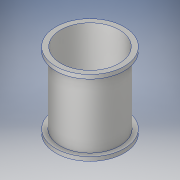
# Autodesk Inventor part: Radiation Sheild 55K
Saved by Autodesk Inventor 2018 (Build 220112000, 112)
## iProperties
Created: 2018-10-10
Part Number: Radiation Sheild 55K
Material: Aluminum 6061
Document SubType Name: Modeling
Designer: freyja
Mass: 27400.2 g
Surface Area: 12721.2 cm^2
Volume: 10148.2 cm^3
Density: 2.7 g/cm^3
Appearance: Aluminum - Flat
Author: freyja
Autodesk Inventor part; units mm, degrees
ref_plane "YZ Plane" through (0, 0, 0) normal (1, 0, 0) x (0, 1, 0)
ref_plane "XZ Plane" through (0, 0, 0) normal (0, 1, 0) x (-1, 0, 0)
ref_plane "XY Plane" through (0, 0, 0) normal (0, 0, 1) x (1, 0, 0)
sketch "Sketch1" plane through (0, 0, 0) normal (0, 1, 0) x (-1, 0, 0)
  circle A0 centre (0, 0) radius 184.15
  circle A1 centre (0, 0) radius 215.9
  dimension "d0" = 368.3
  dimension "d1" = 431.8
  constraints: 2 centre point, 2 coincident
  measures "d0" diameter of A0
  measures "d1" diameter of A1
extrude "Extrusion1" add sketch "Sketch1" along normal blind 25.4
sketch "Sketch2" plane through (0, 25.4, 0) normal (0, 1, 0) x (1, 0, 0)
  circle A0 centre (0, 0) radius 184.15
  circle A1 centre (0, 0) radius 187.96
  dimension "d4" = 368.3
  dimension "d5" = 375.92
  constraints: 2 centre point, 2 coincident
  measures "d4" diameter of A0
  measures "d5" diameter of A1
extrude "Extrusion2" add sketch "Sketch2" along normal blind 423.8625
sketch "Sketch3" plane through (0, 449.2625, 0) normal (0, 1, 0) x (1, 0, 0)
  circle A0 centre (0, 0) radius 184.15
  circle A1 centre (0, 0) radius 215.9
  dimension "d8" = 368.3
  dimension "d9" = 431.8
  constraints: 2 centre point, 2 coincident
  measures "d8" diameter of A0
  measures "d9" diameter of A1
extrude "Extrusion3" add sketch "Sketch3" along normal blind 25.4
body "Solid1"
